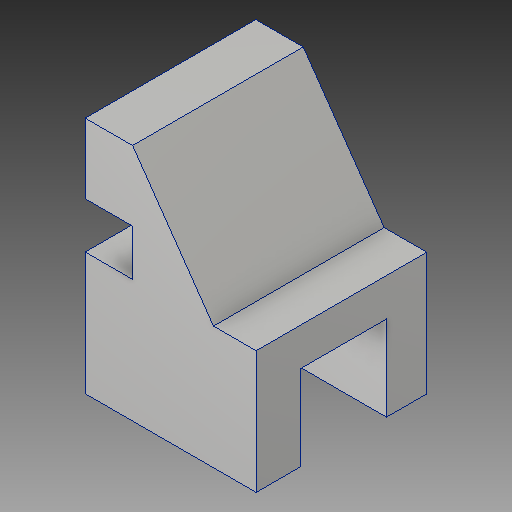
# Autodesk Inventor part: 小虎鉗-左側
Saved by Autodesk Inventor 2017 (Build 210142000, 142)
## iProperties
Part Number: 小虎鉗-左側
Material: 鋁合金 6061
Document SubType Name: Modeling
Designer: user
Density: 2.7 g/cm^3
Appearance: 鋁 - 平面
Author: user
Autodesk Inventor part; units mm, degrees
ref_plane "YZ Plane" through (0, 0, 0) normal (1, 0, 0) x (0, 1, 0)
ref_plane "XZ Plane" through (0, 0, 0) normal (0, 1, 0) x (-1, 0, 0)
ref_plane "XY Plane" through (0, 0, 0) normal (0, 0, 1) x (1, 0, 0)
sketch "草圖1" plane through (0, 0, 0) normal (0, 0, 1) x (1, 0, 0)
  line L0 (0, 0) -> (51.3, 0)
  line L1 (51.3, 0) -> (51.3, 36.8)
  line L2 (51.3, 36.8) -> (38.5, 36.8)
  line L3 (38.5, 36.8) -> (14.22, 71.58)
  line L4 (14.22, 71.58) -> (0, 71.58)
  line L5 (0, 71.58) -> (0, 50.64)
  line L6 (0, 50.64) -> (14.22, 50.64)
  line L7 (14.22, 50.64) -> (14.22, 36.8)
  line L8 (14.22, 36.8) -> (0, 36.8)
  line L9 (0, 0) -> (0, 36.8)
  dimension "d0" = 36.8
  dimension "d1" = 14.22
  dimension "d3" = 13.84
  dimension "d4" = 14.22
  dimension "d5" = 71.58
  dimension "d6" = 51.3
  dimension "d7" = 12.8
  constraints: 20 end point, 5 perpendicular, 3 point on line, 1 horizontal, 1 parallel, 1 vertical
  measures "d0" distance between parallel lines of L0 L2
  measures "d1" distance of L3.end L4.end
  measures "d3" distance of L6.end L7.end
  measures "d4" distance between parallel lines of L9 L7
  measures "d5" distance between parallel lines of L0 L4
  measures "d6" distance of L0.start L0.end
  measures "d7" distance of L1.end L2.end
extrude "擠出1" add sketch "草圖1" along normal blind 51.2
sketch "草圖2" plane through (0, 0, 0) normal (-1, 0, 0) x (0, 0, 1)
  line L0 (0, 0) -> (51.2, 0) projected
  line L1 (12.1, 0) -> (12.1, 25.5)
  line L2 (12.1, 25.5) -> (37.8, 25.5)
  line L3 (37.8, 25.5) -> (37.8, -6.925)
  line L4 (37.8, -6.925) -> (13.9148, -5.9857)
  line L5 (13.9148, -5.9857) -> (12.1, 0)
  line L6 (51.2, 36.8) -> (51.2, 0) projected
  dimension "d10" = 25.7
  dimension "d12" = 13.4
  dimension "d13" = 25.5
  constraints: 10 end point, 2 perpendicular, 1 point on line, 1 vertical
  measures "d10" distance of L1.end L2.end
  measures "d12" distance between parallel lines of L6 L3
  measures "d13" distance between parallel lines of L0 L2
extrude "擠出2" cut sketch "草圖2" against normal up to next
sketch "草圖3" plane through (0, 0, 51.2) normal (0, -1, 0) x (1, 0, 0)
  circle A0 centre (44.3, -7.4) radius 2.5
  line L0 (0, -13.4) -> (51.3, -13.4) projected
  line L1 (51.3, -13.4) -> (51.3, 0) projected
  circle A1 centre (5.9, -7.4) radius 2.5
  point P0 (0, -51.2)
  dimension "d16" = 5
  dimension "d18" = 6
  dimension "d19" = 7
  dimension "d22" = 38.4
  constraints: 2 centre point, 1 horizontal, 2 other
  measures "d16" diameter of A0
  measures "d18" distance from line of A0.centre L0
  measures "d19" distance from line of A0.centre L1
  measures "d22" distance of A0.centre A1.centre
extrude "擠出3" cut sketch "草圖3" against normal blind 12.5
pattern_linear "矩形陣列1" count 2 spacing 39 along (0, 0, -1) of "擠出3"
